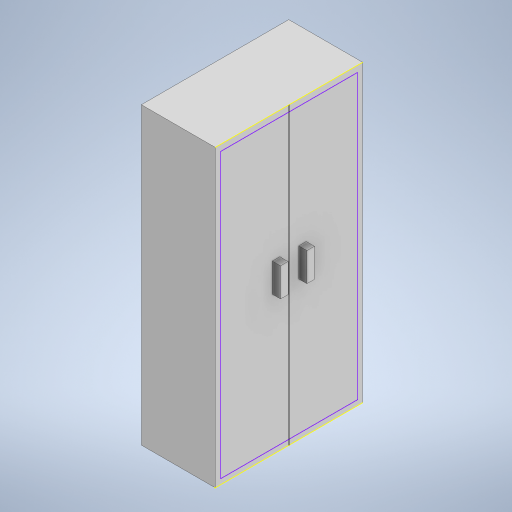
# Autodesk Inventor part: Cabinet
Saved by Autodesk Inventor 2023.2 (Build 272271000, 271)
## iProperties
Created: 2022-12-08
Part Number: Cabinet
Material: Generic
Document SubType Name: Modeling
Designer: Team 4026
Density: 1 g/cm^3
Appearance: Default
Author: Team 4026
Autodesk Inventor part; units mm, degrees
ref_plane "YZ Plane" through (0, 0, 0) normal (1, 0, 0) x (0, 1, 0)
ref_plane "XZ Plane" through (0, 0, 0) normal (0, 1, 0) x (-1, 0, 0)
ref_plane "XY Plane" through (0, 0, 0) normal (0, 0, 1) x (1, 0, 0)
sketch "Sketch2" plane through (0, 0, 0) normal (0, 1, 0) x (-1, 0, 0)
  line L0 (0, 0) -> (457.2, 0)
  line L1 (457.2, 0) -> (457.2, -914.4)
  line L2 (457.2, -914.4) -> (0, -914.4)
  line L3 (0, -914.4) -> (0, 0)
  line L4 (457.2, -457.2) -> (0, -457.2)
  dimension "d2" = 457.2
  dimension "d3" = 914.4
  constraints: 10 end point, 2 midpoint, 2 parallel, 1 horizontal, 1 perpendicular
  measures "d2" distance of L1.end L2.end
  measures "d3" distance of L0.end L1.end
extrude "Extrusion2" add sketch "Sketch2" along normal blind 1828.8
sketch "Sketch3" plane through (0, 0, 0) normal (1, 0, 0) x (0, 0, -1)
  line L0 (914.4, 1828.8) -> (0, 1828.8) projected
  line L1 (457.2, 1828.8) -> (457.2, 0)
  line L2 (914.4, 0) -> (0, 0) projected
  constraints: 2 end point, 2 midpoint
sketch "Sketch4" plane through (0, 0, 0) normal (1, 0, 0) x (0, 0, -1)
  line L0 (355.1544, 1039.5953) -> (401.9558, 1039.5953)
  line L1 (401.9558, 1039.5953) -> (401.9558, 861.75)
  line L2 (401.9558, 861.75) -> (355.1544, 861.75)
  line L3 (355.1544, 861.75) -> (355.1544, 1039.5953)
  line L4 (518.9593, 861.75) -> (565.7607, 861.75)
  line L5 (565.7607, 861.75) -> (565.7607, 1039.5953)
  line L6 (565.7607, 1039.5953) -> (518.9593, 1039.5953)
  line L7 (518.9593, 1039.5953) -> (518.9593, 861.75)
  point P0 (0, 0)
  constraints: 16 end point, 4 parallel, 2 horizontal, 2 perpendicular, 2 point on line
extrude "Extrusion3" add sketch "Sketch4" along normal blind 50.8
sketch "Sketch5" plane through (0, 0, 0) normal (1, 0, 0) x (0, 0, -1)
  line L0 (34.1958, 1790.2512) -> (883.0565, 1790.2512)
  line L1 (883.0565, 1790.2512) -> (883.0565, 32.1843)
  line L2 (883.0565, 32.1843) -> (34.1958, 32.1843)
  line L3 (34.1958, 32.1843) -> (34.1958, 1790.2512)
  point P0 (0, 0)
  constraints: 8 end point, 2 parallel, 1 horizontal, 1 perpendicular
body "Solid2"
